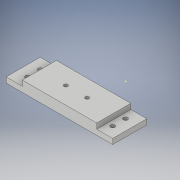
# Autodesk Inventor part: HandleBlock
Saved by Autodesk Inventor 2019 (Build 230136000, 136)
## iProperties
Created: 2020-03-14
Part Number: HandleBlock
Material: Generic
Document SubType Name: Modeling
Designer: james
Density: 1 g/cm^3
Appearance: Default
Author: james
Autodesk Inventor part; units mm, degrees
ref_plane "YZ Plane" through (0, 0, 0) normal (1, 0, 0) x (0, 1, 0)
ref_plane "XZ Plane" through (0, 0, 0) normal (0, 1, 0) x (-1, 0, 0)
ref_plane "XY Plane" through (0, 0, 0) normal (0, 0, 1) x (1, 0, 0)
sketch "Sketch1" plane through (0, 0, 0) normal (0, 1, 0) x (-1, 0, 0)
  line L0 (69.5314, 72.8452) -> (-57.4686, 72.8452)
  line L1 (-57.4686, 72.8452) -> (-57.4686, 32.2052)
  line L2 (-57.4686, 32.2052) -> (69.5314, 32.2052)
  line L3 (69.5314, 32.2052) -> (69.5314, 72.8452)
  point P0 (0, 0)
  dimension "d0" = 127
  dimension "d1" = 40.64
  constraints: 8 end point, 2 parallel, 1 horizontal, 1 perpendicular
  measures "d0" distance of L1.end L2.end
  measures "d1" distance of L2.end L0.start
extrude "Extrusion1" add sketch "Sketch1" along normal blind 6.35
sketch "Sketch2" plane through (0, 6.35, 0) normal (0, 1, 0) x (1, 0, 0)
  line L0 (-50.2274, -32.2052) -> (38.4186, -32.2052)
  line L1 (38.4186, -32.2052) -> (38.4186, -72.8452)
  line L2 (38.4186, -72.8452) -> (-50.2274, -72.8452)
  line L3 (-50.2274, -72.8452) -> (-50.2274, -32.2052)
  line L4 (-69.5314, -32.2052) -> (-69.5314, -72.8452) projected
  line L5 (57.4686, -72.8452) -> (57.4686, -32.2052) projected
  line L6 (57.4686, -32.2052) -> (-69.5314, -32.2052) projected
  line L7 (-69.5314, -72.8452) -> (57.4686, -72.8452) projected
  point P0 (0, 0)
  dimension "d4" = 19.304
  dimension "d5" = 19.05
  dimension "d6" = 0
  dimension "d7" = 0
  constraints: 8 end point, 2 parallel, 1 horizontal, 1 perpendicular
  measures "d4" distance between parallel lines of L4 L3
  measures "d5" distance between parallel lines of L5 L1
  measures "d6" distance between parallel lines of L6 L0
  measures "d7" distance between parallel lines of L7 L2
extrude "Extrusion2" add sketch "Sketch2" along normal blind 6.35 contours L0 L1 L2 L3
sketch "Sketch3" plane through (0, 6.35, 0) normal (0, 1, 0) x (1, 0, 0)
  line L0 (57.4686, -32.2052) -> (38.4186, -32.2052) projected
  line L1 (57.4686, -72.8452) -> (57.4686, -32.2052) projected
  line L2 (-69.5314, -32.2052) -> (-69.5314, -72.8452) projected
  line L3 (-50.2274, -32.2052) -> (-69.5314, -32.2052) projected
  line L4 (-69.5314, -72.8452) -> (-50.2274, -72.8452) projected
  line L5 (38.4186, -72.8452) -> (57.4686, -72.8452) projected
  circle A0 centre (-27.5338, -49.4612) radius 4.3448
  circle A1 centre (16.1358, -48.3961) radius 3.4084
  point P0 (0, 0)
  point P1 (-56.8314, -44.9052)
  point P2 (-56.8314, -60.1452)
  point P3 (44.7686, -44.9052)
  point P4 (44.7686, -60.1452)
  dimension "d10" = 12.7
  dimension "d11" = 12.7
  dimension "d12" = 12.7
  dimension "d13" = 12.7
  dimension "d14" = 12.7
  dimension "d15" = 12.7
  dimension "d16" = 12.7
  dimension "d17" = 12.7
  constraints: 2 centre point
  measures "d10" distance from line of L0 point (44.769, -44.905)
  measures "d11" distance from line of L1 point (44.769, -44.905)
  measures "d12" distance from line of L2 point (-56.831, -44.905)
  measures "d13" distance from line of L3 point (-56.831, -44.905)
  measures "d14" distance from line of L4 point (-56.831, -60.145)
  measures "d15" distance from line of L5 point (44.769, -60.145)
  measures "d16" distance from line of L1 point (44.769, -60.145)
  measures "d17" distance from line of L2 point (-56.831, -60.145)
hole "Hole1" at (-56.8314, 6.35, 44.9052) at (-56.8314, 6.35, 60.1452) at (44.7686, 6.35, 44.9052) at (44.7686, 6.35, 60.1452) direction (0, -1, 0) diameter 5.1054 depth 25.4 tip angle 118 clearance for "Flat Head Machine Screw (82)" size "#10" standard "Ansi Unified Screw Threads"
sketch "Sketch4" plane through (0, 0, 0) normal (0, -1, 0) x (1, 0, 0)
  circle A0 centre (-18.7314, 52.5252) radius 4.445
  circle A1 centre (6.6686, 52.5252) radius 4.445
  line L0 (57.4686, 32.2052) -> (-69.5314, 32.2052) projected
  line L1 (57.4686, 72.8452) -> (57.4686, 32.2052) projected
  line L2 (-69.5314, 32.2052) -> (-69.5314, 72.8452) projected
  point P0 (0, 0)
  dimension "d25" = 20.32
  dimension "d26" = 0
  dimension "d27" = 50.8
  dimension "d28" = 50.8
  dimension "d29" = 8.89
  dimension "d30" = 8.89
  constraints: 2 centre point
  measures "d25" distance from line of L0 A0.centre
  measures "d26" vertical distance of A0.centre A1.centre
  measures "d27" distance from line of L1 A1.centre
  measures "d28" distance from line of L2 A0.centre
  measures "d29" diameter of A0
  measures "d30" diameter of A1
extrude "Extrusion3" cut sketch "Sketch4" against normal blind 7.62
sketch "Sketch5" plane through (0, 0, 0) normal (0, -1, 0) x (1, 0, 0)
  point P0 (0, 0)
sketch "Sketch6" plane through (0, 0, 0) normal (0, -1, 0) x (1, 0, 0)
  circle A0 centre (-18.7314, 52.5252) radius 4.445 projected
  circle A1 centre (6.6686, 52.5252) radius 4.445 projected
  point P0 (0, 0)
  constraints: 2 coincident
hole "Hole2" at (-18.7314, 0, 52.5252) at (6.6686, 0, 52.5252) direction (0, 1, 0) diameter 4.4958 depth 25.4 tip angle 118 clearance for "Flat Head Machine Screw (82)" size "#8" standard "Ansi Unified Screw Threads"
body "Solid1"
